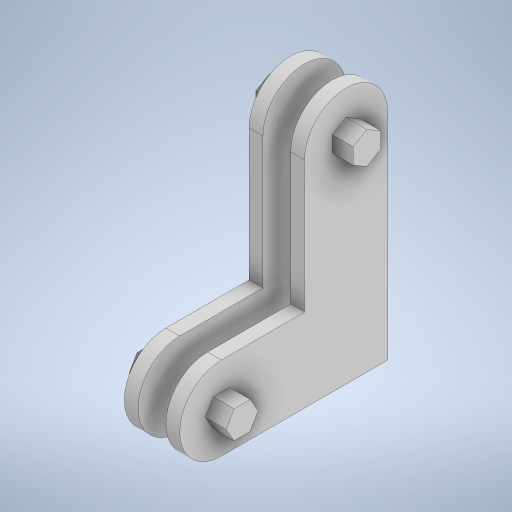
# Autodesk Inventor part: mount_shaft_mount
Saved by Autodesk Inventor 2023 (Build 270158000, 158)
## iProperties
Created: 2023-09-19
Part Number: mount_shaft_mount
Material: Generic
Document SubType Name: Modeling
Designer: Peter
Density: 1 g/cm^3
Appearance: Default
Author: Peter
Autodesk Inventor part; units mm, degrees
ref_plane "XZ Plane" through (0, 0, 0) normal (0, 1, 0) x (-1, 0, 0)
ref_plane "XY Plane" through (0, 0, 0) normal (0, 0, 1) x (1, 0, 0)
sketch "Sketch1" plane through (0, 0, 0) normal (1, 0, 0) x (0, 1, 0)
  arc A0 (120.65, -76.2) -> (120.65, 0) centre (120.65, -38.1) ccw
  arc A1 (0, 76.2) -> (-76.2, 76.2) centre (-38.1, 76.2) ccw
  line L0 (0, 76.2) -> (0, 0)
  line L1 (0, 0) -> (120.65, 0)
  line L2 (120.65, -76.2) -> (-76.2, -76.2)
  line L3 (-76.2, -76.2) -> (-76.2, 76.2)
  dimension "d1" = 76.2
  dimension "d2" = 76.2
  dimension "d7" = 0
  dimension "d8" = 120.65
  dimension "d9" = 0
  dimension "d10" = 76.2
  constraints: 8 end point, 4 point on circle, 4 tangent, 2 centre point, 2 horizontal, 2 vertical
  measures "d1" diameter of A0
  measures "d2" diameter of A1
  measures "d7" distance from line of L0 point (0, 0)
  measures "d8" distance from line of L0 A0.centre
  measures "d9" distance from line of point (0, 0) L1
  measures "d10" distance of L0.start L0.end
extrude "Extrusion1" add sketch "Sketch1" along normal blind 12.7
ref_plane "Work Plane1" through (25.4, 0, 0) normal (1, 0, 0) x (0, 1, 0)
sketch "Sketch2" plane through (0, 0, 0) normal (-1, 0, 0) x (0, 0, 1)
  arc A0 (0, 120.65) -> (-76.2, 120.65) centre (-38.1, 120.65) ccw construction
  arc A1 (76.2, -76.2) -> (76.2, 0) centre (76.2, -38.1) ccw construction
  line L0 (-38.1, 105.9853) -> (-50.8, 113.3177)
  line L1 (-50.8, 113.3177) -> (-50.8, 127.9823)
  line L2 (-50.8, 127.9823) -> (-38.1, 135.3147)
  line L3 (-38.1, 135.3147) -> (-25.4, 127.9823)
  line L4 (-25.4, 127.9823) -> (-25.4, 113.3177)
  line L5 (-25.4, 113.3177) -> (-38.1, 105.9853)
  line L6 (61.5353, -38.1) -> (68.8677, -25.4)
  line L7 (68.8677, -25.4) -> (83.5323, -25.4)
  line L8 (83.5323, -25.4) -> (90.8647, -38.1)
  line L9 (90.8647, -38.1) -> (83.5323, -50.8)
  line L10 (83.5323, -50.8) -> (68.8677, -50.8)
  line L11 (68.8677, -50.8) -> (61.5353, -38.1)
  point P0 (0, 0)
  point P1 (76.2, -50.8)
  point P2 (76.2, -25.4)
  dimension "d12" = 25.4
  dimension "d13" = 25.4
  constraints: 24 end point, 2 coincident, 2 midpoint, 26 other
  measures "d12" distance of point (76.2, -50.8) point (76.2, -25.4)
  measures "d13" distance from line of L0 L3.end
extrude "Extrusion2" add sketch "Sketch2" along normal blind 19.05
mirror "Mirror2" about plane through (25.4, 0, 0) normal (1, 0, 0)
body "Solid1"
